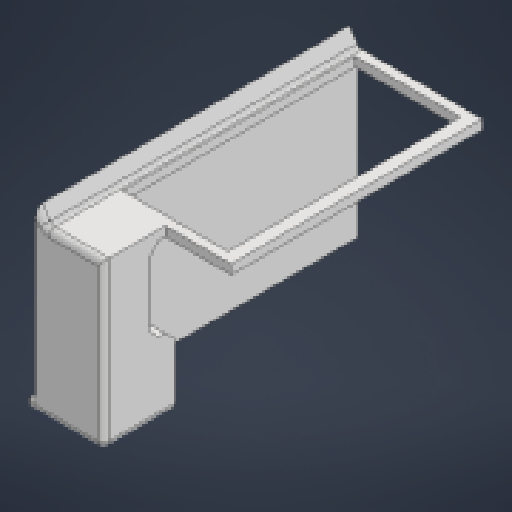
# Autodesk Inventor part: 主体
Saved by Autodesk Inventor 2025 (Build 290162000, 162)
## iProperties
Created: 2025-11-30
Part Number: 主体
Material: 常规
Document SubType Name: Modeling
Designer: XH
Density: 1 g/cm^3
Appearance: 默认
Author: XH
Autodesk Inventor part; units mm, degrees
ref_plane "YZ Plane" through (0, 0, 0) normal (1, 0, 0) x (0, 1, 0)
ref_plane "XZ Plane" through (0, 0, 0) normal (0, 1, 0) x (-1, 0, 0)
ref_plane "XY Plane" through (0, 0, 0) normal (0, 0, 1) x (1, 0, 0)
sketch "草图1" plane through (0, 0, 0) normal (1, 0, 0) x (0, 1, 0)
  line L0 (-22.5, 37.5) -> (22.5, 37.5)
  line L1 (22.5, 37.5) -> (22.5, -37.5)
  line L2 (22.5, -37.5) -> (-22.5, -37.5)
  line L3 (-22.5, -37.5) -> (-22.5, 37.5)
  line L4 (-22.5, 37.5) -> (22.5, -37.5) construction
  line L5 (22.5, 37.5) -> (-22.5, -37.5) construction
  point P0 (0, 0)
  dimension "d2" = 75
  dimension "d3" = 45
  constraints: 12 end point, 2 midpoint, 2 parallel, 1 horizontal, 1 perpendicular
  measures "d2" distance of L2.end L0.start
  measures "d3" distance of L1.end L2.end
extrude "拉伸1" add sketch "草图1" along normal blind 3
sketch "草图2" plane through (3, 0, 0) normal (1, 0, 0) x (0, 0, -1)
  line L0 (37.5, 22.5) -> (-37.5, 22.5) projected
  line L1 (-37.5, 22.5) -> (37.5, 22.5)
  line L2 (37.5, 22.5) -> (37.5, 19.5)
  line L3 (37.5, 19.5) -> (-37.5, 19.5)
  line L4 (-37.5, 19.5) -> (-37.5, 22.5)
  line L5 (37.5, -22.5) -> (37.5, 22.5) projected
  point P0 (0, 0)
  dimension "d4" = 3
  constraints: 8 end point, 2 parallel, 1 collinear, 1 horizontal, 1 perpendicular
  measures "d4" distance between parallel lines of L0 L3
extrude "拉伸2" add sketch "草图2" along normal blind 40
sketch "草图4" plane through (3, 0, 0) normal (1, 0, 0) x (0, 0, -1)
  line L0 (32.5, -7.5) -> (42.5, -7.5)
  line L1 (42.5, -7.5) -> (42.5, 7.5)
  line L2 (42.5, 7.5) -> (32.5, 7.5)
  line L3 (32.5, 7.5) -> (32.5, -7.5)
  line L4 (37.5, -22.5) -> (37.5, 22.5) projected
  line L5 (32.5, -7.5) -> (42.5, 7.5) construction
  line L6 (42.5, -7.5) -> (32.5, 7.5) construction
  point P0 (0, 0)
  point P1 (37.5, 0)
  dimension "d9" = 5
  dimension "d10" = 15
  constraints: 12 end point, 3 midpoint, 2 parallel, 1 horizontal, 1 perpendicular
  measures "d9" distance between parallel lines of L3 L4
  measures "d10" distance of L0.end L1.end
extrude "拉伸4" cut sketch "草图4" against normal blind 11.25
mirror "镜像1" about plane through (0, 0, 0) normal (0, 0, 1) of "拉伸4"
sketch "草图5" plane through (3, 19.5, -37.5) normal (0, -1, 0) x (1, 0, 0)
  point P0 (-3, 37.5)
ref_plane "工作平面1" through (0, 0, 0) normal (0, 0, 1) x (1, 0, 0)
move faces "移动1" translate (0, 0, 3) faces at (15.3333, 21.5, 37.5)
move faces "移动2" translate (0, 0, -3) faces at (15.3333, 21.5, -37.5)
sketch "草图6" plane through (3, 0, 0) normal (1, 0, 0) x (0, 0, -1)
  line L0 (-37.5, -27.5) -> (37.5, -27.5) projected
  line L1 (-37.5, 22.5) -> (-37.5, -27.5) projected
  line L2 (37.5, -27.5) -> (37.5, 22.5) projected
  line L3 (-40.5, 22.5) -> (-40.5, -30.5)
  line L4 (-40.5, -30.5) -> (40.5, -30.5)
  line L5 (40.5, -30.5) -> (40.5, 22.5)
  line L6 (-40.5, -12.5) -> (40.5, -12.5)
  line L7 (-30.5, -30.5) -> (-30.5, -12.5)
  point P0 (0, 0)
  point P1 (37.5, -22.5)
  dimension "d19" = 3
  dimension "d20" = 18
  dimension "d21" = 10
  constraints: 10 end point, 4 point on line, 2 perpendicular, 2 other
  measures "d19" distance between parallel lines of L1 L3
  measures "d20" distance between parallel lines of L4 L6
  measures "d21" distance between parallel lines of L3 L7
ref_plane "工作平面2" through (0, -27.5, -37.5) normal (1, 0, 0) x (0, 1, 0)
extrude "拉伸5" add sketch "草图6" against normal up to surface (3 mm away)
sketch "草图7" plane through (0, 0, 0) normal (-1, 0, 0) x (0, 0, 1)
  line L0 (-37.5, 47.5) -> (37.5, 47.5) projected
  line L1 (-37.5, -27.5) -> (-37.5, 47.5) projected
  line L2 (37.5, -27.5) -> (-37.5, -27.5) projected
  line L3 (37.5, 47.5) -> (37.5, -27.5) projected
  line L4 (-40.5, -30.5) -> (-40.5, 50.5)
  line L5 (-40.5, 50.5) -> (40.5, 50.5)
  line L6 (40.5, 50.5) -> (40.5, -30.5)
  line L7 (40.5, -30.5) -> (-40.5, -30.5)
  line L8 (-37.5, -12.5) -> (-40.5, -12.5) projected
  line L9 (40.5, -12.5) -> (-40.5, -12.5)
  point P0 (0, 0)
  point P1 (37.5, -12.5)
  dimension "d24" = 3
  constraints: 10 end point, 1 collinear, 1 point on line, 3 other
  measures "d24" distance between parallel lines of L2 L7
ref_plane "工作平面3" through (-2, 40.5, -40.5) normal (-1, 0, 0) x (0, 0, 1)
extrude "拉伸6" add sketch "草图7" along normal up to surface (2 mm away) contours L1 L2 L3 L9 L6 L7 L4 L8
sketch "草图8" plane through (3, 19.5, 40.5) normal (0, -1, 0) x (1, 0, 0)
  line L0 (40, -81) -> (40, 0) projected
  line L1 (40, -40.5) -> (0, -40.5)
  line L2 (0, -81) -> (0, 0) projected
  line L3 (2, -78) -> (36, -78)
  line L4 (36, -78) -> (36, -3)
  line L5 (36, -3) -> (2, -3)
  line L6 (2, -3) -> (2, -78)
  line L7 (2, -78) -> (36, -3) construction
  line L8 (36, -78) -> (2, -3) construction
  line L9 (0, -81) -> (40, -81) projected
  point P0 (-3, -40.5)
  point P1 (19, -40.5)
  dimension "d27" = 4
  dimension "d28" = 3
  dimension "d29" = 2
  constraints: 14 end point, 4 midpoint, 2 parallel, 1 horizontal, 1 perpendicular, 1 point on line
  measures "d27" distance between parallel lines of L0 L4
  measures "d28" distance between parallel lines of L9 L3
  measures "d29" distance between parallel lines of L2 L6
extrude "拉伸7" cut sketch "草图8" against normal blind 10 contours L4 L3 L6 L1 | L1 L6 L5 L4
fillet "圆角1" radius 2 1 edges at (3, 19.5, 0)
ref_plane "工作平面4" through (-30, -27.5, -37.5) normal (0, 0, -1) x (0, 1, 0)
sketch "草图9" plane through (-30, -27.5, -37.5) normal (0, 0, -1) x (0, 1, 0)
  point P0 (27.5, 30)
sketch "草图10" plane through (0, 7.5, -40.5) normal (0, 0, -1) x (-1, 0, 0)
  line L0 (0, 15) -> (0, 0) projected
  line L1 (0, 15) -> (0, 19.484)
  line L2 (0, 19.484) -> (-3.2492, 15)
  line L3 (0, 15) -> (-43, 15) projected
  point P0 (0, -7.5)
  constraints: 4 end point, 1 point on line, 1 vertical
extrude "拉伸8" add sketch "草图10" against normal up to surface (81 mm away)
fillet "圆角2" radius 2 1 edges at (3.2492, 22.5, 0)
delete faces "删除1" heal yes whole lump no faces at (1, -9.1667, -37.5) (0.3333, -12.5, -39.5) (1, -9.1667, 37.5) (1, -12.5, 38.5)
sketch "草图11" plane through (3, -30.5, 40.5) normal (1, 0, 0) x (0, 0, -1)
  line L0 (0, 0) -> (81, 0) projected
  line L1 (3, 0) -> (-20, 0)
  line L2 (-20, 0) -> (-20, 50.0098)
  line L3 (-20, 50.0098) -> (3, 50.0098)
  line L4 (3, 50.0098) -> (3, 0)
  line L5 (3, 50) -> (3, 53) projected
  line L6 (0, 23) -> (0, 0) projected
  point P0 (40.5, 30.5)
  point P1 (3, 0)
  dimension "d36" = 20
  constraints: 8 end point, 2 parallel, 1 collinear, 1 horizontal, 1 perpendicular, 1 point on line
  measures "d36" distance between parallel lines of L2 L6
extrude "拉伸9" add sketch "草图11" along normal blind 18.75
delete faces "删除2" heal yes whole lump no faces at (1, 7.5, 36.8333) (2, 2.5, 32.5)
sketch "草图12" plane through (4.2698, 22.5, 40.5) normal (0, 0, 1) x (1, 0, 0)
  line L0 (-6.2698, -30) -> (-4.2698, -30) projected
  line L1 (-6.2698, -30) -> (-6.2698, -53) projected
  line L2 (-1.2698, -53) -> (-6.2698, -53) projected
  line L3 (-1.2698, -2.9902) -> (-1.2698, -53) projected
  line L4 (-1.2698, -2.9902) -> (17.4802, -2.9902) projected
  line L5 (17.4802, -2.9902) -> (17.4802, -3) projected
  line L6 (17.4802, -3) -> (38.7302, -3) projected
  line L7 (38.7302, 0) -> (38.7302, -3) projected
  line L8 (0, 0) -> (38.7302, 0) projected
  arc A0 (-1.6195, 0.8265) -> (0, 0) centre (0, 2) ccw projected
  line L9 (-4.2698, 4.484) -> (-1.6195, 0.8265) projected
  line L10 (-4.2698, -30) -> (-4.2698, 4.484) projected
  line L11 (17.4802, -53) -> (17.4802, -3) projected
  line L12 (17.4802, -3) -> (17.4802, 0)
  point P0 (-4.2698, -22.5)
  constraints: 2 end point, 1 perpendicular, 1 point on line
extrude "拉伸10" add sketch "草图12" along normal up to surface (20 mm away) contours L0 L10 L9 A0 L8 L12 L4 L3 L2 L1
delete faces "删除3" heal yes whole lump no faces at (-0.6667, -14.1667, 37.5)
fillet "圆角3" radius 2 6 edges at (21.75, -4, 60.5) (21.75, -30.5, 49) (9.875, -30.5, 60.5) (3.3607, 22.7186, 60.5) (1.3251, 25.1552, 60.5) (13.0099, 22.5, 60.5)
sketch "草图13" plane through (39, 22.5, 37.5) normal (0, 0, -1) x (-1, 0, 0)
  point P0 (39, -22.5)
sketch "草图14" plane through (21.75, -30.5, 40.5) normal (1, 0, 0) x (0, 0, -1)
  line L0 (-7, 50) -> (18.6513, 50)
  line L1 (18.6513, 50) -> (18.6513, 23)
  line L2 (18.6513, 23) -> (-7, 23)
  line L3 (-7, 23) -> (-7, 50)
  line L4 (3, 2) -> (3, 50) projected
  line L5 (0, 50) -> (81, 50) projected
  point P0 (40.5, 30.5)
  point P1 (3, 48)
  dimension "d43" = 10
  dimension "d46" = 27
  constraints: 8 end point, 2 parallel, 1 collinear, 1 horizontal, 1 perpendicular
  measures "d43" distance between parallel lines of L3 L4
  measures "d46" distance between parallel lines of L2 L0
extrude "拉伸11" cut sketch "草图14" against normal up to surface (18.75 mm away)
chamfer "倒角1" distance 5 angle 45 2 edges at (12.375, -7.5, 47.5) (12.375, 19.5, 47.5)
chamfer "倒角2" distance 3 angle 45 1 edges at (12.375, -7.5, 37.5)
move faces "移动3" translate (0, 0, -2) faces at (15.5, 8.8333, 47.5)
sketch "草图15" plane through (0, 7.5, -40.5) normal (-1, 0, 0) x (0, 0, 1)
  line L0 (0, 0) -> (8, 0) projected
  line L1 (8, -15) -> (0, -15)
  line L2 (0, -15) -> (0, 0)
  line L3 (0, 0) -> (8, 0)
  line L4 (8, 0) -> (8, -15)
  point P0 (40.5, -7.5)
  constraints: 8 end point, 2 parallel, 1 horizontal, 1 perpendicular
extrude "拉伸12" add sketch "草图15" against normal up to surface (3 mm away)
